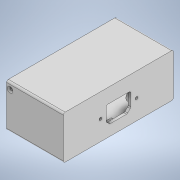
# Autodesk Inventor part: high_voltage_cover
Saved by Autodesk Inventor 2021.3 (Build 253353010, 353A)
## iProperties
Created: 2021-12-08
Part Number: high_voltage_cover
Material: Generic
Document SubType Name: Modeling
Designer: au504769
Density: 1 g/cm^3
Appearance: Default
Author: au504769
## iProperties of the stored document _3DPrint.ipt
Created: 2021-12-09
Part Number: _3DPrint
Material: Generic
Document SubType Name: Modeling
Designer: au504769
Density: 1 g/cm^3
Appearance: Default
Author: au504769
Autodesk Inventor part; units mm, degrees
ref_plane "YZ Plane" through (0, 0, 0) normal (1, 0, 0) x (0, 1, 0)
ref_plane "XZ Plane" through (0, 0, 0) normal (0, 1, 0) x (-1, 0, 0)
ref_plane "XY Plane" through (0, 0, 0) normal (0, 0, 1) x (1, 0, 0)
sketch "Sketch1" plane through (0, 0, 0) normal (1, 0, 0) x (0, 1, 0)
  line L0 (0, 0) -> (48, 0)
  line L1 (48, 0) -> (48, -122)
  line L2 (48, -122) -> (0, -122)
  line L3 (0, -122) -> (0, 0)
  line L4 (3, -3) -> (45, -3)
  line L5 (45, -3) -> (45, -119)
  line L6 (45, -119) -> (3, -119)
  line L7 (3, -119) -> (3, -3)
  line L8 (45, -6.2) -> (6.2, -6.2)
  line L9 (6.2, -6.2) -> (6.2, -115.8)
  line L10 (6.2, -115.8) -> (45, -115.8)
  line L11 (42, -6.2) -> (42, -115.8)
  line L12 (45, -3) -> (45, 0) construction
  line L13 (45, -3) -> (48, -3) construction
  line L14 (45, -119) -> (45, -122) construction
  line L15 (3, -3) -> (0, -3) construction
  line L16 (42, -6.2) -> (42, -3) construction
  line L17 (42, -59.8864) -> (45, -61) construction
  line L18 (6.2, -6.2) -> (3, -6.2) construction
  line L19 (42, -115.8) -> (42, -119) construction
  dimension "d0" = 116
  dimension "d1" = 42
  dimension "d2" = 3
  dimension "d3" = 3.2
  dimension "d5" = 3
  constraints: 40 end point, 12 perpendicular, 12 point on line, 6 equal length, 4 parallel, 3 horizontal, 1 midpoint
  measures "d0" distance between parallel lines of L6 L4
  measures "d1" distance between parallel lines of L7 L5
  measures "d2" distance between parallel lines of L0 L4
  measures "d3" distance between parallel lines of L4 L8
  measures "d5" distance between parallel lines of L5 L11
extrude "Extrusion1" add sketch "Sketch1" along normal blind 3 contours L0 L1 L2 L3 | L4 L5 L8 L9 L10 L6 L7 | L5 L10 L11 L8 | L11 L10 L9 L8
extrude "Extrusion2" add sketch "Sketch1" against normal blind 60
extrude "Extrusion3" add sketch "Sketch1" against normal blind 49 contours L5 L10 L11 L8
extrude "Extrusion4" add sketch "Sketch1" against normal blind 35 contours L4 L5 L8 L9 L10 L6 L7
sketch "Sketch2" plane through (-60, 3, -3) normal (0, 1, 0) x (1, 0, 0)
  line L0 (25, 3.2) -> (25, 112.8) projected
  line L1 (25, 6.5) -> (21.1, 6.5)
  arc A0 (21.1, 10.5) -> (21.1, 6.5) centre (21.1, 8.5) ccw
  line L2 (21.1, 10.5) -> (25, 10.5)
  line L3 (25, 10.5) -> (25, 6.5)
  line L4 (25, 0) -> (25, 116) projected
  line L5 (25, 109.5) -> (25, 105.5)
  line L6 (25, 105.5) -> (21.1, 105.5)
  arc A1 (21.1, 109.5) -> (21.1, 105.5) centre (21.1, 107.5) ccw
  line L7 (21.1, 109.5) -> (25, 109.5)
  line L8 (25, 105.5) -> (25, 10.5) construction
  line L9 (25, 109.5) -> (25, 112.8) construction
  line L10 (25, 6.5) -> (25, 3.2) construction
  point P0 (60, -3)
  point P1 (25, 109.5)
  dimension "d14" = 4
  dimension "d15" = 99
  dimension "d16" = 3.9
  constraints: 18 end point, 4 point on circle, 4 point on line, 4 tangent, 3 collinear, 3 equal length, 3 horizontal, 2 centre point, 2 perpendicular
  measures "d14" distance between parallel lines of L2 L1
  measures "d15" distance of A0.centre A1.centre
  measures "d16" distance from line of L0 A0.centre
extrude "Extrusion5" [suppressed]
sketch "Sketch10" plane through (3, 0, 0) normal (1, 0, 0) x (0, 0, -1)
  point P0 (0, 0)
sketch "Sketch11" plane through (3, 0, 0) normal (1, 0, 0) x (0, 0, -1)
  line L0 (52.0784, 12) -> (69.9216, 12)
  line L1 (74.75, 16.8284) -> (74.75, 30)
  line L2 (72.75, 32) -> (49.25, 32)
  line L3 (47.25, 30) -> (47.25, 16.8284)
  line L4 (50.6642, 12.5858) -> (47.8358, 15.4142)
  line L5 (71.3358, 12.5858) -> (74.1642, 15.4142)
  arc A0 (49.25, 32) -> (47.25, 30) centre (49.25, 30) ccw
  arc A1 (74.75, 30) -> (72.75, 32) centre (72.75, 30) ccw
  arc A2 (74.1642, 15.4142) -> (74.75, 16.8284) centre (72.75, 16.8284) ccw
  arc A3 (69.9216, 12) -> (71.3358, 12.5858) centre (69.9216, 14) ccw
  arc A4 (50.6642, 12.5858) -> (52.0784, 12) centre (52.0784, 14) ccw
  arc A5 (47.25, 16.8284) -> (47.8358, 15.4142) centre (49.25, 16.8284) ccw
  circle A6 centre (41, 22) radius 1.5
  circle A7 centre (81, 22) radius 1.5
  line L6 (47.25, 34.8284) -> (47.25, 23.4142) construction
  line L7 (47.25, 12) -> (47.25, 23.4142) construction
  line L8 (0, 48) -> (0, 0) construction
  line L9 (122, 48) -> (0, 48) construction
  line L10 (79.2679, 25) -> (82.7321, 25)
  line L11 (82.7321, 25) -> (84.4641, 22)
  line L12 (84.4641, 22) -> (82.7321, 19)
  line L13 (82.7321, 19) -> (79.2679, 19)
  line L14 (79.2679, 19) -> (77.5359, 22)
  line L15 (79.2679, 25) -> (77.5359, 22)
  line L16 (81, 22) -> (79.2679, 25) construction
  line L17 (81, 22) -> (82.7321, 25) construction
  line L18 (81, 22) -> (79.2679, 19) construction
  line L19 (81, 22) -> (84.4641, 22) construction
  circle A8 centre (81, 22) radius 5.75
  circle A9 centre (41, 22) radius 5.75
  line L20 (39.2679, 25) -> (42.7321, 25)
  line L21 (42.7321, 25) -> (44.4641, 22)
  line L22 (44.4641, 22) -> (42.7321, 19)
  line L23 (42.7321, 19) -> (39.2679, 19)
  line L24 (39.2679, 19) -> (37.5359, 22)
  line L25 (37.5359, 22) -> (39.2679, 25)
  line L26 (44.4641, 22) -> (41, 22) construction
  line L27 (41, 22) -> (37.5359, 22) construction
  line L28 (61, 32) -> (0, 32) construction
  line L29 (61, 32) -> (122, 32) construction
  line L30 (122, 0) -> (122, 48) construction
  line L31 (41, 22) -> (47.25, 22) construction
  line L32 (81, 22) -> (74.75, 22) construction
  point P0 (74.75, 12)
  point P1 (51.25, 12)
  point P2 (47.25, 16)
  point P3 (70.75, 12)
  point P4 (74.75, 16)
  dimension "d65" = 4
  dimension "d66" = 4
  dimension "d67" = 4
  dimension "d68" = 4
  dimension "d69" = 20
  dimension "d70" = 27.5
  dimension "d71" = 2
  dimension "d72" = 40
  dimension "d73" = 3
  dimension "d81" = 6
  dimension "d82" = 11.5
  dimension "d110" = 26
  dimension "d111" = 16
  constraints: 60 end point, 19 point on line, 18 equal length, 12 point on circle, 12 tangent, 10 centre point, 8 parallel, 7 equal radius, 7 horizontal, 4 collinear, 2 coincident, 2 midpoint, 2 perpendicular, 1 vertical alignment
  measures "d65" distance of point (51.25, 12) L7.start
  measures "d66" distance of point (47.25, 16) L7.start
  measures "d67" distance of point (70.75, 12) point (74.75, 12)
  measures "d68" distance of point (74.75, 16) point (74.75, 12)
  measures "d69" distance between parallel lines of L2 L0
  measures "d70" distance between parallel lines of L1 L3
  measures "d71" radius of A0
  measures "d72" distance of L16.start A6.centre
  measures "d73" diameter of A6
  measures "d81" distance between parallel lines of L13 L10
  measures "d82" diameter of A8
  measures "d110" distance from line of L9 A6.centre
  measures "d111" distance between parallel lines of L9 L2
extrude "Extrusion8" cut sketch "Sketch11" against normal up to surface (3 mm away) contours A4 L4 A5 L3 A0 L2 A1 L1 A2 L5 A3 L0 | A6 | A7
extrude "Extrusion10" add sketch "Sketch11" against normal blind 6 contours A8 | A9
ref_plane "Work Plane2" through (-35, 42, -61) normal (0, 0, 1) x (1, 0, 0)
ref_plane "Work Plane3" through (-60, 22.5, -3) normal (0, 1, 0) x (1, 0, 0)
sketch "Sketch13" plane through (-35, 42, -61) normal (0, 0, 1) x (1, 0, 0)
  line L0 (35, 0) -> (25, 0) construction
  line L1 (35, 0) -> (35, -10) construction
  line L2 (35, -10) -> (25, 0)
  line L3 (35, -31.8) -> (27, -35.8)
  line L4 (27, -35.8) -> (35, -35.8) construction
  line L5 (35, -35.8) -> (35, -31.8) construction
  point P0 (35, -42)
  dimension "d85" = 10
  dimension "d86" = 10
  dimension "d87" = 4
  dimension "d88" = 8
  constraints: 12 end point, 2 horizontal, 1 coincident, 1 perpendicular, 1 vertical
  measures "d85" distance of L0.start L0.end
  measures "d86" distance of L0.start L1.end
  measures "d87" distance of L4.end L3.start
  measures "d88" distance of L3.end L4.end
sketch "Sketch14" plane through (-60, 22.5, -3) normal (0, 1, 0) x (1, 0, 0)
  line L0 (60, 3.2) -> (35, 3.2) construction
  line L1 (35, 3.2) -> (60, 30.2)
  line L2 (60, 30.2) -> (60, 3.2) construction
  point P0 (60, -3)
  dimension "d101" = 27
  dimension "d102" = 25
  constraints: 6 end point, 1 horizontal, 1 vertical
  measures "d101" distance of L1.end L0.start
  measures "d102" distance of L0.start L0.end
extrude "Rib3" add sketch "Sketch14" along normal mid plane 2 rib yes fills toward (47.5367, 16.666) open curves L1
mirror "Mirror1" about plane through (-35, 42, -61) normal (0, 0, 1) of "Rib3"
extrude "Rib1" add sketch "Sketch13" along normal mid plane 2 rib yes fills toward (30.0354, -4.9646) open curves L2
extrude "Rib2" add sketch "Sketch13" along normal mid plane 2 rib yes fills toward (31.0224, -33.8447) open curves L3
fillet "Fillet1" radius 2 4 edges at (-17.5, 6.2, -115.8) (-47.5, 3, -119) (-17.5, 6.2, -6.2) (-47.5, 3, -3)
fillet "Fillet3" radius 2 4 edges at (-28.5, 48, -122) (-28.5, 0, -122) (-28.5, 0, 0) (-28.5, 48, 0)
fillet "Fillet4" radius 2 10 edges at (-12.5, 23.5, -6.2) (-12.5, 21.5, -6.2) (-4, 6.2, -60) (-4, 6.2, -62) (-5, 42, -62) (-5, 42, -60) (-12.5, 21.5, -115.8) (-12.5, 23.5, -115.8) (-17.5, 42, -115.8) (-17.5, 42, -6.2)
sketch "Sketch6" plane through (0, 0, 0) normal (0, 0, 1) x (1, 0, 0)
  line L0 (-35, 45) -> (-35, 5) projected
  line L1 (-35, 45) -> (-60, 45) projected
  point P0 (0, 0)
  point P1 (-56, 41)
  dimension "d42" = 4
  dimension "d43" = 21
  measures "d42" distance from line of point (-56, 41) L1
  measures "d43" distance from line of L0 point (-56, 41)
sketch "Sketch7" plane through (-60, 0, -2) normal (0, -1, 0) x (1, 0, 0)
  line L0 (22, -108.5) -> (22, -120) construction
  line L1 (63, -120) -> (0, -120) construction
  line L2 (22, -9.5) -> (22, 2) construction
  line L3 (0, 2) -> (63, 2) construction
  line L4 (25, -3) -> (25, -115) construction
  point P0 (60, 2)
  dimension "d33" = 99
  dimension "d34" = 3
  constraints: 4 end point, 3 point on line, 1 collinear, 1 vertical, 1 vertical alignment
  measures "d33" distance of L2.start L0.start
  measures "d34" distance from line of L4 L0.start
hole "Hole1" at (-38, 0, -110.5) at (-38, 0, -11.5) direction (0, 1, 0) diameter 3.4 depth 3 tip angle 118 countersink diameter 6.3 countersink angle 90 clearance for "Countersunk Flat Head Screw DIN EN ISO 2009" size "M3" standard "DIN"
hole "Hole2" at (-56, 41, 0) direction (0, 0, -1) diameter 3.4 depth 3 tip angle 118 countersink diameter 6.3 countersink angle 90 clearance for "Countersunk Flat Head Screw DIN EN ISO 2009" size "M3" standard "DIN"
sketch "Sketch9" plane through (3, 2, -122) normal (0, 0, -1) x (-1, 0, 0)
  circle A0 centre (59, 39) radius 3.15 projected
  point P0 (3, -2)
  constraints: 1 coincident
hole "Hole4" at (-56, 41, -122) direction (0, 0, 1) diameter 3.4 depth 3 tip angle 118 countersink diameter 6.3 countersink angle 90 clearance for "Countersunk Flat Head Screw DIN EN ISO 2009" size "M3" standard "DIN"
sketch "Sketch4" plane through (0, 0, 0) normal (0, 1, 0) x (-1, 0, 0)
  line L0 (-3, 0) -> (-3, -122) projected
  line L1 (60, 0) -> (-3, 0) projected
  line L2 (-3, -122) -> (31, -122)
  line L3 (31, -122) -> (31, 0)
  line L4 (31, 0) -> (-3, 0)
  line L5 (-3, 0) -> (-3, -122)
  point P0 (0, 0)
  point P1 (60, -122)
  dimension "d20" = 34
  constraints: 8 end point, 2 parallel, 1 horizontal, 1 perpendicular, 1 point on line
  measures "d20" distance between parallel lines of L0 L3
extrude "3D_print_test_cut_1" [suppressed]
sketch "Sketch12" plane through (0, 0, 0) normal (0, 1, 0) x (-1, 0, 0)
  line L0 (-3, -122) -> (60, -122) projected
  line L1 (-3, 0) -> (60, 0) projected
  line L2 (60, -122) -> (2, -122)
  line L3 (2, -122) -> (2, 0)
  line L4 (2, 0) -> (60, 0)
  line L5 (60, 0) -> (60, -122)
  line L6 (-3, -2) -> (-3, -120) projected
  point P0 (0, 0)
  dimension "d78" = 5
  constraints: 8 end point, 2 parallel, 1 horizontal, 1 perpendicular, 1 point on line
  measures "d78" distance between parallel lines of L6 L3
extrude "3D_print_test_cut_2" [suppressed]
ref_plane "Work Plane4" through (-56, 41, -145.4545) normal (-1, 0, 0) x (0, 0, 1)
equation "\"d66\" = d65"
equation "\"d67\" = d65"
equation "\"d68\" = d67"
body "Solid1"
